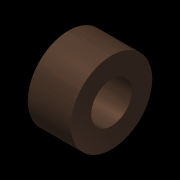
# Autodesk Inventor part: Ball Shifting Outline
Saved by Autodesk Inventor 2014 SP1 (Build 180222100, 222)
## iProperties
Created: 2014-01-10
Part Number: Ball Shifting Outline
Material: Bronze, Cast
Document SubType Name: Modeling
Designer: Rauhul Varma
Density: 8.87 g/cm^3
Appearance: Bronze - Satin
Mass: 5.67233 g
Surface Area: 5.92848 cm^2
Volume: 0.639497 cm^3
Author: Rauhul Varma
Autodesk Inventor part; units mm, degrees
ref_plane "YZ Plane" through (0, 0, 0) normal (1, 0, 0) x (0, 1, 0)
ref_plane "XZ Plane" through (0, 0, 0) normal (0, 1, 0) x (-1, 0, 0)
ref_plane "XY Plane" through (0, 0, 0) normal (0, 0, 1) x (1, 0, 0)
sketch "Sketch1" plane through (0, 0, 0) normal (0, 0, 1) x (1, 0, 0)
  line L0 (0, 0) -> (8.7313, 0) construction
  line L1 (0, 0) -> (0, 7.9375) construction
  line L2 (0, 7.9375) -> (8.7312, 7.9375) construction
  line L3 (8.7312, 7.9375) -> (8.7313, 0) construction
  line L4 (8.7312, 7.9375) -> (45.2438, 7.9375) construction
  line L5 (8.7312, 7.9375) -> (8.7312, 14.2875) construction
  line L6 (8.7312, 14.2875) -> (9.525, 14.2875) construction
  line L7 (9.525, 14.2875) -> (9.525, 0) construction
  line L8 (9.525, 0) -> (8.7313, 0) construction
  line L9 (9.525, 0) -> (19.05, 0) construction
  line L10 (19.05, 0) -> (19.05, 26.67) construction
  line L11 (19.05, 26.67) -> (9.525, 26.67) construction
  line L12 (9.525, 26.67) -> (9.525, 14.2875) construction
  line L13 (14.2875, 0) -> (14.2875, 26.67) construction
  line L14 (14.2875, 17.4625) -> (21.4312, 17.4625) construction
  line L15 (21.4312, 17.4625) -> (21.4313, 0) construction
  line L16 (21.4313, 0) -> (19.05, 0) construction
  line L17 (21.4313, 0) -> (22.225, 0) construction
  line L18 (22.225, 0) -> (22.225, 14.2875) construction
  line L19 (22.225, 14.2875) -> (21.4313, 14.2875) construction
  line L20 (21.4313, 14.2875) -> (21.4313, 0) construction
  line L21 (22.225, 0) -> (31.75, 0) construction
  line L22 (31.75, 0) -> (31.75, 20.32) construction
  line L23 (31.75, 20.32) -> (22.225, 20.32) construction
  line L24 (22.225, 20.32) -> (22.225, 0) construction
  line L25 (26.9875, 20.32) -> (26.9875, 0) construction
  line L26 (26.9875, 17.4625) -> (34.1313, 17.4625) construction
  line L27 (34.1313, 17.4625) -> (34.1313, 0) construction
  line L28 (34.1313, 0) -> (31.75, 0) construction
  line L29 (34.1313, 0) -> (34.925, 0) construction
  line L30 (34.925, 0) -> (34.925, 14.2875) construction
  line L31 (34.925, 14.2875) -> (34.1313, 14.2875) construction
  line L32 (34.1313, 14.2875) -> (34.1313, 0) construction
  line L33 (34.925, 0) -> (36.5125, 0) construction
  line L34 (36.5125, 0) -> (36.5125, 9.525) construction
  line L35 (36.5125, 9.525) -> (34.925, 9.525) construction
  line L36 (34.925, 9.525) -> (34.925, 0) construction
  line L37 (45.2438, 7.9375) -> (45.2438, 0) construction
  line L38 (45.2438, 0) -> (36.5125, 0) construction
  line L39 (11.9063, 26.67) -> (11.9063, 0) construction
  line L40 (24.6063, 20.32) -> (24.6063, 0) construction
  line L41 (0, 7.9375) -> (0, 17.4625) construction
  line L42 (0, 17.4625) -> (8.7312, 17.4625) construction
  line L43 (8.7312, 17.4625) -> (8.7312, 14.2875) construction
  line L44 (0, 3.175) -> (45.2438, 3.175) construction
  circle A0 centre (11.9063, 5.5562) radius 2.3813 construction
  circle A1 centre (24.6063, 5.5562) radius 2.3812 construction
  circle A2 centre (11.9063, 5.8103) radius 2.3813 construction
  circle A3 centre (11.9063, 7.5565) radius 2.3813 construction
  circle A4 centre (24.6063, 5.8103) radius 2.3812 construction
  circle A5 centre (24.6063, 7.5565) radius 2.3812 construction
  line L45 (9.525, 8.1915) -> (14.2875, 8.1915) construction
  line L46 (12.6386, 3.175) -> (14.6388, 5.1753) construction
  line L47 (14.6388, 5.1753) -> (21.8737, 5.1753) construction
  line L48 (21.8737, 5.1753) -> (23.8739, 3.175) construction
  line L49 (22.225, 8.1915) -> (26.9875, 8.1915) construction
  line L50 (10.3187, 5.1753) -> (17.4901, 5.1753) construction
  line L51 (26.1938, 5.1753) -> (19.0224, 5.1753) construction
  line L52 (0, 6.35) -> (6.731, 6.35) construction
  line L53 (6.731, 6.35) -> (6.731, 3.175) construction
  line L54 (10.3187, 5.1753) -> (8.3185, 3.175) construction
  line L55 (17.4901, 5.1753) -> (19.4903, 3.175) construction
  line L56 (19.4903, 3.175) -> (26.1938, 3.175) construction
  line L57 (26.1938, 3.175) -> (28.1015, 0) construction
  line L58 (26.1938, 5.1753) -> (28.194, 3.175) construction
  line L59 (28.194, 3.175) -> (34.8974, 3.175) construction
  line L60 (34.8974, 3.175) -> (36.8052, 0) construction
  line L61 (6.731, 5.5562) -> (45.2438, 5.5563) construction
  line L62 (37.202, 0) -> (33.8635, 5.5563) construction
  line L63 (19.0224, 5.1753) -> (17.0222, 3.175) construction
  line L64 (17.0222, 3.175) -> (-3.175, 3.175) construction
  line L65 (45.2438, 7.9375) -> (45.2438, 17.4625) construction
  line L66 (45.2438, 17.4625) -> (36.5125, 17.4625) construction
  line L67 (36.5125, 17.4625) -> (36.5125, 9.525) construction
  line L68 (45.2438, 7.9375) -> (51.5938, 7.9375) construction
  line L69 (51.5938, 7.9375) -> (51.5938, 0) construction
  line L70 (51.5938, 0) -> (45.2438, 0) construction
  line L71 (51.5938, 6.35) -> (64.2938, 6.35) construction
  line L72 (64.2938, 6.35) -> (64.2938, 0) construction
  line L73 (64.2938, 0) -> (51.5938, 0) construction
  line L74 (-8.1534, 3.175) -> (-8.1534, 2.3812) construction
  line L75 (-8.1534, 0) -> (36.8052, 0) construction
  line L76 (-3.175, 3.175) -> (-3.175, 2.3812) construction
  line L77 (-3.175, 2.3812) -> (-8.1534, 2.3812) construction
  line L78 (-8.1534, 3.175) -> (-8.1534, 6.35) construction
  line L79 (-8.1534, 6.35) -> (-3.175, 6.35) construction
  line L80 (-3.175, 6.35) -> (-3.175, 3.175) construction
  line L81 (-3.175, 0) -> (-3.175, 2.3812) construction
  line L82 (-0.7937, 0) -> (-0.7938, 11.1125) construction
  line L83 (-0.7938, 11.1125) -> (-3.175, 11.1125) construction
  line L84 (-3.175, 11.1125) -> (-3.175, 6.35) construction
  line L85 (-3.175, 3.175) -> (-8.1534, 3.175) construction
  line L86 (-8.1534, 2.3812) -> (-8.1534, 0) construction
  line L87 (-8.1534, 2.7051) -> (-9.652, 2.7051) construction
  line L88 (-9.652, 2.7051) -> (-9.652, 0) construction
  line L89 (-9.652, 0) -> (-8.1534, 0) construction
  line L90 (-8.1534, 1.4224) -> (-5.6134, 1.4224) construction
  line L91 (-5.6134, 1.4224) -> (-5.6134, 0) construction
  line L92 (-5.6134, 1.4224) -> (-3.0734, 1.4224) construction
  line L93 (-3.0734, 1.4224) -> (-3.0734, 0) construction
  line L94 (-3.175, 11.1125) -> (-13.4938, 11.1125) construction
  line L95 (-13.4938, 11.1125) -> (-13.4937, 5.9531) construction
  line L96 (-13.4937, 5.9531) -> (-18.5801, 5.9531) construction
  line L97 (-18.5801, 5.9531) -> (-18.5801, 0) construction
  line L98 (-18.5801, 0) -> (-9.652, 0) construction
  line L99 (-8.1534, 3.9687) -> (-14.6113, 3.9687) construction
  line L100 (-14.6113, 3.9687) -> (-14.6113, 0) construction
  line L101 (-14.6113, 3.429) -> (-10.4457, 3.429) construction
  line L102 (-10.4457, 3.429) -> (-10.4457, 0) construction
  line L103 (-16.9926, 3.175) -> (-16.9926, 0) construction
  line L104 (-16.9926, 3.175) -> (-18.5801, 3.175) construction
  line L105 (6.731, 3.175) -> (6.731, 0) construction
  dimension "d0" = 8.7312
  dimension "d1" = 7.9375
  dimension "d2" = 0.7937
  dimension "d3" = 14.2875
  dimension "d4" = 9.525
  dimension "d5" = 26.67
  dimension "d6" = 7.1437
  dimension "d7" = 17.4625
  dimension "d8" = 0.7937
  dimension "d9" = 14.2875
  dimension "d10" = 9.525
  dimension "d11" = 20.32
  dimension "d12" = 7.1437
  dimension "d13" = 17.4625
  dimension "d14" = 0.7937
  dimension "d15" = 14.2875
  dimension "d16" = 1.5875
  dimension "d17" = 9.525
  dimension "d18" = 8.7312
  dimension "d19" = 2.3813
  dimension "d20" = 2.3813
  dimension "d21" = 17.4625
  dimension "d22" = 3.175
  dimension "d23" = 4.7625
  dimension "d24" = 4.7625
  dimension "d26" = 0.254
  dimension "d28" = 45
  dimension "d29" = 45
  dimension "d30" = 0.254
  dimension "d31" = 7.2348
  dimension "d32" = 5.1753
  dimension "d33" = 7.1713
  dimension "d34" = 1.5875
  dimension "d35" = 7.1713
  dimension "d36" = 1.5875
  dimension "d37" = 6.35
  dimension "d39" = 45
  dimension "d40" = 45
  dimension "d41" = 1.5875
  dimension "d42" = 59
  dimension "d43" = 6.7034
  dimension "d44" = 6.7034
  dimension "d45" = 5.5563
  dimension "d46" = 0.3969
  dimension "d47" = 1.5875
  dimension "d48" = 6.731
  dimension "d52" = 17.4625
  dimension "d53" = 6.35
  dimension "d54" = 12.7
  dimension "d55" = 6.35
  dimension "d56" = 2.3813
  dimension "d57" = 4.9784
  dimension "d58" = 6.35
  dimension "d66" = 2.3813
  dimension "d67" = 0.7937
  dimension "d68" = 11.1125
  dimension "d69" = 2.7051
  dimension "d70" = 1.4986
  dimension "d71" = 1.4224
  dimension "d72" = 2.54
  dimension "d73" = 2.54
  dimension "d74" = 3.9688
  dimension "d75" = 4.1656
  dimension "d76" = 3.429
  constraints: 210 end point, 55 perpendicular, 39 point on line, 34 parallel, 8 collinear, 8 horizontal, 6 centre point, 6 tangent, 4 equal radius, 4 midpoint, 1 symmetric about line, 1 vertical, 12 other
  measures "d0" distance of L0.start L0.end
  measures "d1" distance of L0.start L1.end
  measures "d2" distance of L5.end L6.end
  measures "d3" distance between parallel lines of L8 L6
  measures "d4" distance of L7.end L9.end
  measures "d5" distance of L9.end L10.end
  measures "d6" distance of L14.start L14.end
  measures "d7" distance between parallel lines of L16 L14
  measures "d8" distance of L18.end L19.end
  measures "d9" distance of L17.end L18.end
  measures "d10" distance of L22.end L23.end
  measures "d11" distance between parallel lines of L21 L23
  measures "d12" distance of L26.start L26.end
  measures "d13" distance between parallel lines of L21 L26
  measures "d14" distance of L31.end L30.end
  measures "d15" distance of L29.end L30.end
  measures "d16" distance of L35.end L34.end
  measures "d17" distance of L33.end L34.end
  measures "d18" distance from line of L4.end L34
  measures "d19" distance between parallel lines of L13 L39
  measures "d20" distance between parallel lines of L25 L40
  measures "d21" distance between parallel lines of L0 L42
  measures "d23" diameter of A0
  measures "d24" diameter of A1
  measures "d26" distance between parallel lines of L4 L45
  measures "d28" angle to the sketch x axis of L46
  measures "d29" angle to the sketch x axis of L48
  measures "d30" distance between parallel lines of L49 L4
  measures "d31" distance of L46.end L47.end
  measures "d32" distance between parallel lines of L9 L47
  measures "d33" distance of L50.start L50.end
  measures "d34" distance from line of L50.start L39
  measures "d35" distance of L51.start L51.end
  measures "d36" distance from line of L51.start L40
  measures "d37" distance between parallel lines of L0 L52
  measures "d39" angle to the sketch x axis of L54
  measures "d40" angle to the sketch x axis of L55
  measures "d41" distance from line of L40 L56.end
  measures "d42" angle of L21 L57
  measures "d43" distance of L58.end L59.end
  measures "d44" distance of L55.end L56.end
  measures "d45" distance between parallel lines of L38 L61
  measures "d46" distance of L60.end L62.start
  measures "d47" distance from line of L53 L54.end
  measures "d48" distance between parallel lines of L1 L53
  measures "d52" distance between parallel lines of L38 L66
  measures "d53" distance between parallel lines of L37 L69
  measures "d54" distance of L72.end L69.end
  measures "d55" distance between parallel lines of L73 L71
  measures "d56" distance between parallel lines of L75 L77
  measures "d57" distance between parallel lines of L74 L76
  measures "d58" distance between parallel lines of L75 L79
  measures "d66" distance between parallel lines of L82 L84
  measures "d67" distance between parallel lines of L41 L82
  measures "d68" distance between parallel lines of L75 L83
  measures "d69" distance between parallel lines of L75 L87
  measures "d70" distance of L87.start L87.end
  measures "d71" distance between parallel lines of L75 L90
  measures "d72" distance of L90.start L90.end
  measures "d73" distance of L90.end L92.end
  measures "d74" distance between parallel lines of L98 L99
  measures "d75" distance between parallel lines of L100 L102
  measures "d76" distance between parallel lines of L98 L101
sketch "Sketch2" plane through (0, 0, 0) normal (0, 0, 1) x (1, 0, 0)
  line L0 (0, 6.35) -> (6.731, 6.35) projected
  line L1 (6.731, 6.35) -> (6.731, 3.175) projected
  line L2 (0, 6.35) -> (0, 3.175)
  line L3 (0, 3.175) -> (6.731, 3.175)
  line L4 (-35.1549, 0) -> (80.8685, 0) projected
  point P0 (0, 0)
  constraints: 4 end point, 1 parallel, 1 perpendicular
revolve "Revolution1" add sketch "Sketch2" angle 360 about axis through (-10, 0, 0) along (1, 0, 0)
equation "\"d9\" = d3"
equation "\"d12\" = d6"
equation "\"d13\" = d7"
equation "\"d15\" = d9"
equation "\"d18\" = d0"
equation "\"d20\" = d19"
equation "\"d35\" = d33"
equation "\"d36\" = d34"
equation "\"d43\" = d44"
equation "\"d52\" = d13"
body "Solid1"
